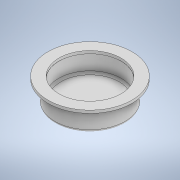
# Autodesk Inventor part: Boat Handle Base
Saved by Autodesk Inventor 2021 (Build 250183000, 183)
## iProperties
Created: 2020-09-02
Part Number: Boat Handle Base
Material: Generic
Document SubType Name: Modeling
Designer: cmzgt
Density: 1 g/cm^3
Appearance: Default
Author: cmzgt
## iProperties of the stored document _3DPrint.ipt
Created: 2020-09-02
Part Number: _3DPrint
Material: Generic
Document SubType Name: Modeling
Designer: cmzgt
Density: 1 g/cm^3
Appearance: Default
Author: cmzgt
Autodesk Inventor part; units mm, degrees
ref_plane "YZ Plane" through (0, 0, 0) normal (1, 0, 0) x (0, 1, 0)
ref_plane "XZ Plane" through (0, 0, 0) normal (0, 1, 0) x (-1, 0, 0)
ref_plane "XY Plane" through (0, 0, 0) normal (0, 0, 1) x (1, 0, 0)
sketch "Sketch1" plane through (0, 0, 0) normal (0, 1, 0) x (-1, 0, 0)
  circle A0 centre (0, 0) radius 26.543
  dimension "d0" = 53.086
  constraints: 1 centre point, 1 coincident
  measures "d0" diameter of A0
extrude "Extrusion1" add sketch "Sketch1" along normal blind 16.3068
sketch "Sketch2" plane through (0, 16.3068, 0) normal (0, 1, 0) x (1, 0, 0)
  circle A0 centre (0, 0) radius 23.495
  dimension "d3" = 46.99
  constraints: 1 centre point, 1 coincident
  measures "d3" diameter of A0
extrude "Extrusion2" cut sketch "Sketch2" against normal blind 12.7
sketch "Sketch3" plane through (0, 16.3068, 0) normal (0, 1, 0) x (1, 0, 0)
  circle A0 centre (0, 0) radius 31.623
  circle A1 centre (0, 0) radius 23.401
  dimension "d6" = 63.246
  constraints: 2 centre point, 2 coincident
  measures "d6" diameter of A0
extrude "Extrusion4" add sketch "Sketch3" along normal blind 2.1082
fillet "Fillet1" radius 2.032 1 edges at (26.543, 0, 0)
fillet "Fillet2" radius 1.524 1 edges at (-23.495, 3.6068, 0)
body "Solid1"
